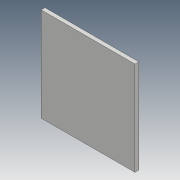
# Autodesk Inventor part: tapa
Saved by Autodesk Inventor 2017 (Build 210142000, 142)
## iProperties
Created: 2020-06-11
Part Number: tapa
Material: Generic
Document SubType Name: Modeling
Designer: c
Density: 1 g/cm^3
Appearance: Default
Author: c
Autodesk Inventor part; units mm, degrees
ref_plane "YZ Plane" through (0, 0, 0) normal (1, 0, 0) x (0, 1, 0)
ref_plane "XZ Plane" through (0, 0, 0) normal (0, 1, 0) x (-1, 0, 0)
ref_plane "XY Plane" through (0, 0, 0) normal (0, 0, 1) x (1, 0, 0)
sketch "Sketch1" plane through (0, 0, 0) normal (0, 1, 0) x (-1, 0, 0)
  line L0 (12, 19) -> (-37, 19)
  line L1 (-37, 19) -> (-37, -30)
  line L2 (-37, -30) -> (12, -30)
  line L3 (12, -30) -> (12, 19)
  point P0 (0, 0)
  dimension "d0" = 49
  dimension "d1" = 49
  constraints: 8 end point, 2 parallel, 1 horizontal, 1 perpendicular
  measures "d0" distance of L2.end L1.end
  measures "d1" distance of L1.end L0.end
extrude "Extrusion1" add sketch "Sketch1" along normal blind 2
body "Solid1"
